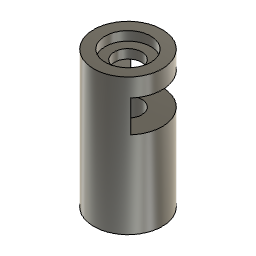
_corner stand.2b617d94-af73-4d40-9075-9734b86fe06d (Autodesk Fusion 360 design; units mm, degrees)
Autodesk Fusion 360 part; units mm, degrees
sketch "Sketch1" plane through (0, 0, 0) normal (0, 0, 1) x (1, 0, 0)
  circle A0 centre (0, 0) radius 7.5
  dimension "d1" = 15
  constraint coincident A0.centre origin
  measures "d1" diameter of A0
extrude "Extrude1" add sketch "Sketch1" along normal blind 30
sketch "Sketch2" plane through (0, 0, 30) normal (0, 0, 1) x (-1, 0, 0)
  circle A0 centre (0, 0) radius 7.5
  line L0 (0, 0) -> (-10.0601, 0)
  line L1 (-10.0601, 0) -> (-10.0601, -9.4901)
  line L2 (-10.0601, -9.4901) -> (0, -9.4901)
  line L3 (0, -9.4901) -> (0, 0)
  constraint horizontal L0
  constraint vertical L1
  constraint horizontal L2
  constraint vertical L3
  constraint coincident A0.centre L0.start
sketch "Sketch3" plane through (0, 0, 30) normal (0, 0, 1) x (-1, 0, 0)
  circle A0 centre (0, 0) radius 7.5
  circle A1 centre (0, 0) radius 5
  dimension "d8" = 10
  constraint coincident A0.centre A1.centre
  measures "d8" diameter of A1
extrude "Extrude4" cut sketch "Sketch3" against normal blind 2 contours A1
sketch "Sketch4" plane through (0, 0, 28) normal (0, 0, 1) x (-1, 0, 0)
  circle A0 centre (0, 0) radius 5
  circle A1 centre (0, 0) radius 3
  dimension "d11" = 6
  constraint coincident A0.centre A1.centre
  measures "d11" diameter of A1
extrude "Extrude5" cut sketch "Sketch4" against normal blind 2 contours A1
sketch "Sketch5" plane through (0, 0, 26) normal (0, 0, 1) x (-1, 0, 0)
  circle A0 centre (0, 0) radius 3
  line L0 (-8, -8) -> (5, -8)
  line L1 (5, -8) -> (5, 5)
  line L2 (5, 5) -> (-8, 5)
  line L3 (-8, 5) -> (-8, -8)
  line L4 (-8, -8) -> (5, 5) construction
  line L5 (5, -8) -> (-8, 5) construction
  point P0 (-1.5, -1.5)
  constraint horizontal L0
  constraint perpendicular L0 L1
  constraint parallel L0 L2
  constraint parallel L1 L3
  constraint coincident L4 P0
  constraint coincident L5 P0
extrude "Extrude6" cut sketch "Sketch5" against normal blind 7 contours A0 | L0 L1 L2 L3
sketch "Sketch6" plane through (0, 0, 19) normal (0, 0, 1) x (-1, 0, 0)
  arc A0 (-5.5902, 5) -> (5, -5.5902) centre (0, 0) ccw
  line L0 (5, -5.5902) -> (5, 5)
  line L1 (5, 5) -> (-5.5902, 5)
  circle A1 centre (0, 0) radius 3
  dimension "d16" = 6
  constraint coincident A0.centre A1.centre
  measures "d16" diameter of A1
extrude "Extrude7" cut sketch "Sketch6" against normal blind 10 contours A1
